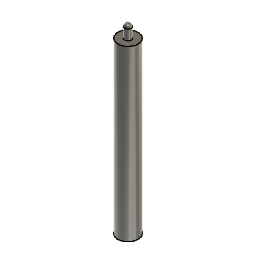
column (Autodesk Fusion 360 design; units mm, degrees)
Autodesk Fusion 360 part; units mm, degrees
cylinder "CylinderPrimitive1" add diameter 6 height 50 placed x (1, 0, 0) y (0, 1, 0) z (0, 0, 1) at (0, 0, 0)
cylinder "CylinderPrimitive2" add diameter 2 height 3 placed x (1, 0, 0) y (0, 1, 0) z (0, 0, 1) at (0, 0, 50)
extrude "Extrude1" add 1 faces at (-0.3296, 0.5031, 53) along direction (0, 0, 1) blind 1
fillet "Fillet1" radius 1 1 faces at (-0.3296, 0.5031, 54)
cylinder "CylinderPrimitive3" cut diameter 2 height -5 placed x (0, 1, 0) y (1, 0, 0) z (0, 0, -1) at (0, 0, 0)
